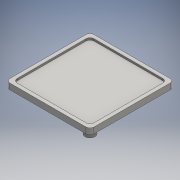
# Autodesk Inventor part: Controller Mount
Saved by Autodesk Inventor 2016 (Build 200138000, 138)
## iProperties
Created: 2016-10-22
Part Number: Controller Mount
Material: Generic
Document SubType Name: Modeling
Designer: Kurtis
Density: 1 g/cm^3
Appearance: Default
Author: Kurtis
Autodesk Inventor part; units mm, degrees
ref_plane "YZ Plane" through (0, 0, 0) normal (1, 0, 0) x (0, 1, 0)
ref_plane "XZ Plane" through (0, 0, 0) normal (0, 1, 0) x (-1, 0, 0)
ref_plane "XY Plane" through (0, 0, 0) normal (0, 0, 1) x (1, 0, 0)
sketch "Sketch Base" plane through (0, 0, 0) normal (0, 0, 1) x (1, 0, 0)
  line L0 (0, 0) -> (36, 0)
  line L1 (36, 0) -> (36, 36)
  line L2 (36, 36) -> (0, 36)
  line L3 (0, 36) -> (0, 0)
  line L4 (0, 0) -> (36, 36) construction
  line L5 (36, 0) -> (0, 36) construction
  line L6 (3, 3) -> (33, 3) construction
  line L7 (33, 3) -> (33, 33) construction
  line L8 (33, 33) -> (3, 33) construction
  line L9 (3, 33) -> (3, 3) construction
  line L10 (3, 3) -> (33, 33) construction
  line L11 (33, 3) -> (3, 33) construction
  circle A0 centre (3, 33) radius 1.5
  circle A1 centre (33, 3) radius 1.5
  circle A2 centre (3, 33) radius 2.5
  circle A3 centre (33, 3) radius 2.5
  line L12 (-1, -1) -> (37, -1)
  line L13 (37, -1) -> (37, 37)
  line L14 (37, 37) -> (-1, 37)
  line L15 (-1, 37) -> (-1, -1)
  line L16 (-1, -1) -> (37, 37) construction
  line L17 (37, -1) -> (-1, 37) construction
  line L18 (-3, -3) -> (39, -3)
  line L19 (39, -3) -> (39, 39)
  line L20 (39, 39) -> (-3, 39)
  line L21 (-3, 39) -> (-3, -3)
  line L22 (-3, -3) -> (39, 39) construction
  line L23 (39, -3) -> (-3, 39) construction
  point P0 (18, 18)
  dimension "d0" = 36
  dimension "d1" = 36
  dimension "d2" = 30
  dimension "d3" = 30
  dimension "d4" = 3
  dimension "d6" = 3
  dimension "d8" = 5
  dimension "d11" = 5
  dimension "d12" = 38
  dimension "d13" = 38
  dimension "d14" = 42
  dimension "d15" = 42
  constraints: 48 end point, 8 parallel, 7 midpoint, 4 centre point, 4 coincident, 4 horizontal, 4 perpendicular
  measures "d0" distance of L2.end L1.end
  measures "d1" distance of L1.end L0.end
  measures "d2" distance of L8.end L7.end
  measures "d3" distance of L7.end L6.end
  measures "d4" diameter of A0
  measures "d6" diameter of A1
  measures "d8" diameter of A2
  measures "d11" diameter of A3
  measures "d12" distance of L14.end L13.end
  measures "d13" distance of L13.end L12.end
  measures "d14" distance of L20.end L19.end
  measures "d15" distance of L19.end L18.end
extrude "Extrusion1" add sketch "Sketch Base" against normal blind 5 contours A2 | A3
extrude "Extrusion5" add sketch "Sketch Base" along normal blind 2 contours L3 L2 L1 L0 | A0 | A1 | A2 | A3 | L15 L14 L13 L12 | L21 L20 L19 L18
sketch "Sketch2" plane through (0, 0, 2) normal (0, 0, 1) x (1, 0, 0)
  line L0 (-3, 39) -> (-3, -3) projected
  line L1 (39, -3) -> (39, 39) projected
  line L2 (-3, -3) -> (39, -3)
  line L3 (39, -3) -> (39, 39)
  line L4 (39, 39) -> (-3, 39)
  line L5 (-3, 39) -> (-3, -3)
  line L6 (-3, -3) -> (39, 39) construction
  line L7 (-1.2, -1.2) -> (37.2, -1.2)
  line L8 (37.2, -1.2) -> (37.2, 37.2)
  line L9 (37.2, 37.2) -> (-1.2, 37.2)
  line L10 (-1.2, 37.2) -> (-1.2, -1.2)
  line L11 (-1.2, -1.2) -> (37.2, 37.2) construction
  line L12 (37.2, -1.2) -> (-1.2, 37.2) construction
  point P0 (0, 0)
  point P1 (18, 18)
  dimension "d30" = 38.4
  dimension "d31" = 38.4
  constraints: 22 end point, 4 parallel, 3 midpoint, 2 horizontal, 2 perpendicular
  measures "d30" distance of L9.end L8.end
  measures "d31" distance of L8.end L7.end
extrude "Extrusion8" add sketch "Sketch2" along normal blind 1
fillet "Fillet1" radius 2 8 edges at (-3, -3, 1.5) (-3, 39, 1.5) (39, 39, 1.5) (39, -3, 1.5) (-1.2, 37.2, 2.5) (37.2, 37.2, 2.5) (37.2, -1.2, 2.5) (-1.2, -1.2, 2.5)
fillet "Fillet2" radius 2 2 edges at (0.5, 33, 0) (30.5, 3, 0)
body "Solid1"
